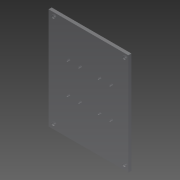
# Autodesk Inventor part: YBedPlate
Saved by Autodesk Inventor 2014 SP1 (Build 180222100, 222)
## iProperties
Created: 2013-12-28
Part Number: YBedPlate
Material: Wood (Birch)
Document SubType Name: Modeling
Designer: Jack
Density: 0.55 g/cm^3
Appearance: Birch - Natural Polished
Author: Jack
Autodesk Inventor part; units mm, degrees
ref_plane "YZ Plane" through (0, 0, 0) normal (1, 0, 0) x (0, 1, 0)
ref_plane "XZ Plane" through (0, 0, 0) normal (0, 1, 0) x (-1, 0, 0)
ref_plane "XY Plane" through (0, 0, 0) normal (0, 0, 1) x (1, 0, 0)
sketch "Sketch1" plane through (0, 0, 0) normal (0, 1, 0) x (-1, 0, 0)
  line L0 (0, 0) -> (256, 0)
  line L1 (256, 0) -> (256, 326)
  line L2 (256, 326) -> (0, 326)
  line L3 (0, 326) -> (0, 0)
  dimension "d0" = 256
  dimension "d1" = 326
  constraints: 8 end point, 2 perpendicular, 1 horizontal, 1 parallel
  measures "d0" distance of L0.start L0.end
  measures "d1" distance of L0.end L1.end
extrude "Extrusion1" add sketch "Sketch1" along normal blind 10
sketch "Sketch2" plane through (0, 10, 0) normal (0, 1, 0) x (1, 0, 0)
  line L0 (0, 0) -> (-256, 0) projected
  line L1 (0, -326) -> (0, 0) projected
  circle A0 centre (-196.7, -212) radius 2.25
  circle A1 centre (-59.3, -212) radius 2.25
  circle A2 centre (-96.7, -212) radius 2.25
  circle A3 centre (-159.3, -212) radius 2.25
  circle A4 centre (-196.7, -114) radius 2.25
  circle A5 centre (-59.3, -114) radius 2.25
  circle A6 centre (-96.7, -114) radius 2.25
  circle A7 centre (-159.3, -114) radius 2.25
  dimension "d4" = 4.5
  dimension "d5" = 4.5
  dimension "d6" = 4.5
  dimension "d7" = 4.5
  dimension "d8" = 4.5
  dimension "d9" = 4.5
  dimension "d10" = 4.5
  dimension "d11" = 4.5
  dimension "d12" = 98
  dimension "d13" = 137.4
  dimension "d14" = 37.4
  dimension "d15" = 37.4
  dimension "d16" = 114
  dimension "d17" = 59.3
  constraints: 8 centre point, 6 horizontal alignment, 4 vertical alignment
  measures "d4" diameter of A0
  measures "d5" diameter of A1
  measures "d6" diameter of A2
  measures "d7" diameter of A3
  measures "d8" diameter of A4
  measures "d9" diameter of A5
  measures "d10" diameter of A6
  measures "d11" diameter of A7
  measures "d12" distance of A1.centre A5.centre
  measures "d13" distance of A0.centre A1.centre
  measures "d14" distance of A0.centre A3.centre
  measures "d15" distance of A2.centre A1.centre
  measures "d16" distance from line of L0 A5.centre
  measures "d17" distance from line of L1 A5.centre
extrude "Extrusion2" cut sketch "Sketch2" against normal blind 10
sketch "Sketch3" plane through (0, 0, 0) normal (0, -1, 0) x (1, 0, 0)
  line L0 (0, 0) -> (-256, 0) projected
  line L1 (0, 326) -> (0, 0) projected
  line L2 (-256, 326) -> (0, 326) projected
  line L3 (-256, 0) -> (-256, 326) projected
  circle A0 centre (-242, 312) radius 2.65
  circle A1 centre (-14, 312) radius 2.65
  circle A2 centre (-14, 14) radius 2.65
  circle A3 centre (-242, 14) radius 2.65
  dimension "d20" = 5.3
  dimension "d21" = 5.3
  dimension "d22" = 5.3
  dimension "d23" = 5.3
  dimension "d24" = 14
  dimension "d25" = 14
  dimension "d26" = 14
  dimension "d27" = 14
  constraints: 4 centre point, 2 horizontal alignment, 2 vertical alignment
  measures "d20" diameter of A0
  measures "d21" diameter of A1
  measures "d22" diameter of A2
  measures "d23" diameter of A3
  measures "d24" distance from line of L2 A0.centre
  measures "d25" distance from line of L3 A0.centre
  measures "d26" distance from line of L1 A2.centre
  measures "d27" distance from line of L0 A2.centre
extrude "Extrusion3" cut sketch "Sketch3" against normal blind 10 contours A0 | A1 | A2 | A3
sketch "Sketch4" plane through (0, 0, 0) normal (0, -1, 0) x (1, 0, 0)
  circle A0 centre (-14, 14) radius 2.65 projected
  circle A1 centre (-242, 312) radius 2.65 projected
  circle A2 centre (-14, 312) radius 2.65 projected
  circle A3 centre (-242, 14) radius 2.65 projected
  circle A4 centre (-242, 312) radius 5
  circle A5 centre (-14, 312) radius 5
  circle A6 centre (-14, 14) radius 5
  circle A7 centre (-242, 14) radius 5
  dimension "d30" = 10
  dimension "d31" = 10
  dimension "d32" = 10
  dimension "d33" = 10
  constraints: 4 centre point, 4 coincident
  measures "d30" diameter of A4
  measures "d31" diameter of A5
  measures "d32" diameter of A6
  measures "d33" diameter of A7
extrude "Extrusion4" cut sketch "Sketch4" against normal blind 4
body "Solid1"
